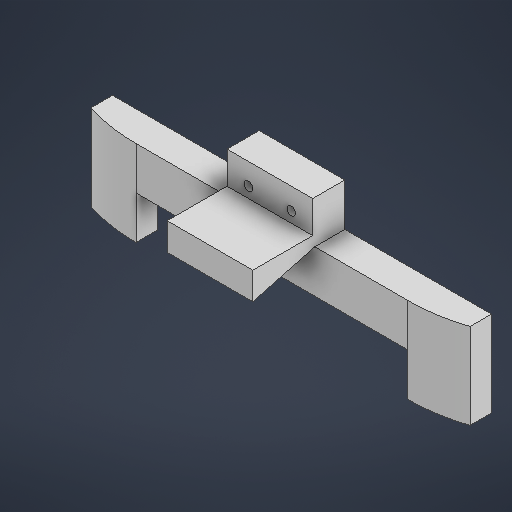
# Autodesk Inventor part: 라이다 고정
Saved by Autodesk Inventor 2026.2 (Build 302298000, 298)
## iProperties
Created: 2025-11-27
Part Number: 라이다 고정
Material: 일반
Document SubType Name: Modeling
Designer: PC
Density: 1 g/cm^3
Appearance: 기본값
Author: PC
Autodesk Inventor part; units mm, degrees
ref_plane "YZ Plane" through (0, 0, 0) normal (1, 0, 0) x (0, 1, 0)
ref_plane "XZ Plane" through (0, 0, 0) normal (0, 1, 0) x (-1, 0, 0)
ref_plane "XY Plane" through (0, 0, 0) normal (0, 0, 1) x (1, 0, 0)
sketch "스케치1" plane through (0, 0, 0) normal (0, 1, 0) x (-1, 0, 0)
  line L0 (124.1226, 0) -> (-124.1226, 0) projected
  line L1 (0, -98.3487) -> (0, 29.2174) projected
  line L2 (63.5, 0) -> (-63.5, 0)
  arc A0 (88.5, -4) -> (63.5, 0) centre (63.5, -80.125) ccw
  line L3 (63.5, 0) -> (63.5, 10)
  line L4 (88.5, -4) -> (88.5, 6)
  arc A1 (88.5, 6) -> (63.5, 10) centre (63.5, -70.125) ccw
  line L5 (63.5, 10) -> (0, 10)
  arc A2 (-63.5, 0) -> (-88.5, -4) centre (-63.5, -80.125) ccw
  line L6 (-63.5, 0) -> (-63.5, 10)
  line L7 (-88.5, -4) -> (-88.5, 6)
  arc A3 (-63.5, 10) -> (-88.5, 6) centre (-63.5, -70.125) ccw
  point P0 (0, 0)
  dimension "d0" = 127
  dimension "d1" = 10
  dimension "d2" = 10
  dimension "d3" = 14
  dimension "d4" = 25
  constraints: 12 end point, 8 point on circle, 5 symmetric about line, 4 centre point, 2 tangent, 2 vertical, 1 horizontal, 1 midpoint, 1 perpendicular, 1 point on line, 2 other
  measures "d0" distance of L2.start L2.end
  measures "d1" distance of L2.start L3.end
  measures "d2" distance of L4.start L4.end
  measures "d3" vertical distance of L3.end L4.start
  measures "d4" distance between parallel lines of L3 L4
extrude "돌출1" add sketch "스케치1" along normal blind 20 contours L4 A0 L0 | A2 L7 L0 | L0 L7 A3 L6 | L0 L3 A1 L4
sketch "스케치2" plane through (0, 20, 0) normal (0, 1, 0) x (1, 0, 0)
  point P0 (0, 0)
sketch "스케치3" plane through (0, 20, 0) normal (0, 1, 0) x (1, 0, 0)
  line L0 (-63.5, -10) -> (-63.5, 0) projected
  arc A0 (-88.5, 4) -> (-63.5, 0) centre (-63.5, 80.125) ccw projected
  line L1 (-88.5, 4) -> (-88.5, -6) projected
  arc A1 (-88.5, -6) -> (-63.5, -10) centre (-63.5, 70.125) ccw projected
  line L2 (88.5, -6) -> (88.5, 4) projected
  arc A2 (63.5, 0) -> (88.5, 4) centre (63.5, 80.125) ccw projected
  line L3 (63.5, 0) -> (63.5, -10) projected
  arc A3 (63.5, -10) -> (88.5, -6) centre (63.5, 70.125) ccw projected
  line L4 (-63.5, -10) -> (63.5, -10)
  line L5 (63.5, -10) -> (63.5, 0)
  line L6 (63.5, 0) -> (-63.5, 0)
  line L7 (-63.5, 0) -> (-63.5, -10)
  line L8 (-88.5, 4) -> (88.5, 4)
  point P0 (0, 0)
  constraints: 10 end point, 2 horizontal, 2 parallel, 1 perpendicular
extrude "돌출2" add sketch "스케치3" along normal blind 20
sketch "스케치4" plane through (0, 0, 0) normal (1, 0, 0) x (0, 1, 0)
  line L0 (40, 10) -> (32.2354, 38.9778)
  line L1 (40, 6) -> (40, 10) projected
  line L2 (40, -4) -> (60, -4)
  line L3 (32.2354, 38.9778) -> (45, 38.9778)
  line L4 (40, 6) -> (40, -4) projected
  line L5 (45, 38.9778) -> (45, 11)
  line L6 (60, 11) -> (60, -4)
  line L7 (0, 6) -> (40, 6) projected
  line L8 (60, 11) -> (45, 11)
  point P0 (0, 0)
  point P1 (20, 10)
  dimension "d9" = 165
  dimension "d11" = 30
  dimension "d12" = 20
  dimension "d13" = 5
  dimension "d16" = 15
  constraints: 12 end point, 3 horizontal, 1 vertical
  measures "d9" angle of L1 L0
  measures "d11" distance of L0.start L0.end
  measures "d12" distance of L2.start L2.end
  measures "d13" distance from line of L3.end L4
  measures "d16" distance between parallel lines of L2 L8
extrude "돌출3" add sketch "스케치4" along normal mid plane 40
sketch "스케치5" plane through (88.5, 20, -4) normal (0, 0, -1) x (-1, 0, 0)
  line L0 (0, 0) -> (177, 0) projected
  line L1 (177, 0) -> (177, 20) projected
  line L2 (108.5, 20) -> (177, 20) projected
  line L3 (108.5, 40) -> (108.5, 20) projected
  line L4 (108.5, 40) -> (68.5, 40) projected
  line L5 (68.5, 20) -> (68.5, 40) projected
  line L6 (0, 20) -> (68.5, 20) projected
  line L7 (0, 0) -> (0, 20) projected
  line L8 (68.5, 30) -> (108.5, 30)
  circle A0 centre (78.5056, 30) radius 2
  circle A1 centre (98.5056, 30) radius 2
  point P0 (88.5, -20)
  dimension "d17" = 4
  dimension "d18" = 4
  dimension "d19" = 20
  constraints: 2 centre point, 2 end point, 2 midpoint, 2 point on line
  measures "d17" diameter of A0
  measures "d18" diameter of A1
  measures "d19" distance of A1.centre A0.centre
extrude "돌출4" cut sketch "스케치5" against normal blind 40 contours A0 L8 | L8 A0 | A1 L8 | L8 A1
sketch "스케치6" plane through (88.5, 20, -4) normal (0, 0, -1) x (-1, 0, 0)
  circle A0 centre (78.5056, 30) radius 2 projected
  circle A1 centre (98.5056, 30) radius 2 projected
  circle A2 centre (78.5056, 30) radius 4
  circle A3 centre (98.5056, 30) radius 4
  point P0 (88.5, -20)
  dimension "d22" = 8
  dimension "d23" = 8
  constraints: 2 centre point, 2 coincident
  measures "d22" diameter of A2
  measures "d23" diameter of A3
extrude "돌출5" cut sketch "스케치6" against normal blind 4 contours A0 | A2 | A3
